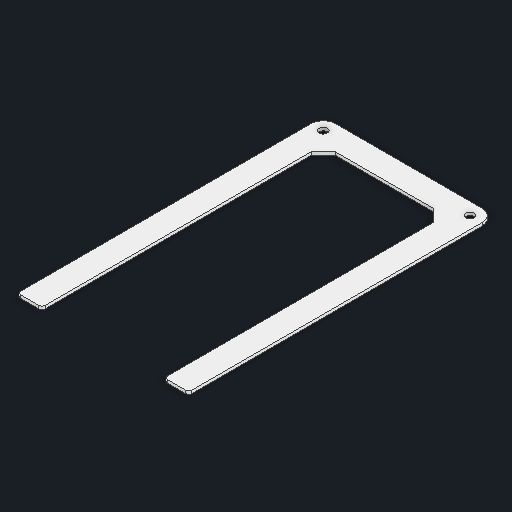
# Autodesk Inventor part: Ring Guard
Saved by Autodesk Inventor 2025.1 (Build 291241000, 241)
## iProperties
Created: 2025-01-02
Part Number: Ring Guard
Material: Acetal Resin, White
Document SubType Name: Modeling
Designer: avere
Density: 1.425 g/cm^3
Appearance: Smooth - White
Author: avere
Autodesk Inventor part; units mm, degrees
ref_plane "YZ Plane" through (0, 0, 0) normal (1, 0, 0) x (0, 1, 0)
ref_plane "XZ Plane" through (0, 0, 0) normal (0, 1, 0) x (-1, 0, 0)
ref_plane "XY Plane" through (0, 0, 0) normal (0, 0, 1) x (1, 0, 0)
sketch "Sketch1" plane through (0, 0, 0) normal (0, 1, 0) x (-1, 0, 0)
  circle A0 centre (-36.9127, -68.2201) radius 2.1844
  circle A1 centre (39.2873, -68.2201) radius 2.1844
  arc A2 (39.2873, -74.5701) -> (45.6373, -68.2201) centre (39.2873, -68.2201) ccw
  arc A3 (-43.2627, -68.2201) -> (-36.9127, -74.5701) centre (-36.9127, -68.2201) ccw
  line L0 (39.2873, -74.5701) -> (-36.9127, -74.5701)
  line L1 (-43.2627, -68.2201) -> (-43.2627, 82.5924)
  line L2 (45.6373, -68.2201) -> (45.6373, 82.5924)
  line L3 (32.9373, 82.5924) -> (32.9373, -55.5201)
  line L4 (-30.5627, -55.5201) -> (-30.5627, 82.5924)
  line L5 (-32.1502, 84.1799) -> (-41.6752, 84.1799)
  line L6 (44.0498, 84.1799) -> (34.5248, 84.1799)
  arc A4 (45.6373, 82.5924) -> (44.0498, 84.1799) centre (44.0498, 82.5924) ccw
  arc A5 (34.5248, 84.1799) -> (32.9373, 82.5924) centre (34.5248, 82.5924) ccw
  arc A6 (-30.5627, 82.5924) -> (-32.1502, 84.1799) centre (-32.1502, 82.5924) ccw
  arc A7 (-41.6752, 84.1799) -> (-43.2627, 82.5924) centre (-41.6752, 82.5924) ccw
  line L7 (26.5873, -61.8701) -> (-24.2127, -61.8701)
  line L8 (32.9373, -55.5201) -> (26.5873, -61.8701)
  line L9 (-30.5627, -55.5201) -> (-24.2127, -61.8701)
  point P0 (0, 0)
  point P1 (-43.2627, 84.1799)
  point P2 (45.6373, 84.1799)
  point P3 (-30.5627, -61.8701)
  point P4 (32.9373, -61.8701)
  dimension "d0" = 152.4
  dimension "d1" = 152.4
  dimension "d2" = 1.5875
  dimension "d3" = 6.35
  dimension "d4" = 6.35
  dimension "d5" = 6.35
  dimension "d6" = 6.35
  constraints: 20 end point, 12 point on circle, 8 centre point, 8 point on line, 8 tangent, 3 equal radius, 3 horizontal, 3 vertical, 2 coincident, 2 perpendicular, 1 parallel, 2 other
  measures "d0" distance of L1.start point (-43.263, 84.18)
  measures "d1" distance of L2.start point (45.637, 84.18)
  measures "d2" radius of A4
  measures "d3" distance of L8.start point (32.937, -61.87)
  measures "d4" distance of L7.start point (32.937, -61.87)
  measures "d5" distance of L9.start point (-30.563, -61.87)
  measures "d6" distance of L9.end point (-30.563, -61.87)
extrude "Extrusion1" add sketch "Sketch1" along normal blind 1.5875
equation "\"d4\" = d3"
equation "\"d5\" = d3"
equation "\"d6\" = d5"
body "Solid1"
